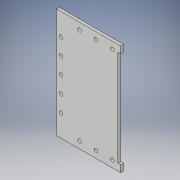
# Autodesk Inventor part: КВ33.000.103 - Стенка тонкая
Saved by Autodesk Inventor 2019 (Build 230136000, 136)
## iProperties
Created: 2021-04-18
Part Number: КВ33.000.103 - Стенка тонкая
Material: Типовые
Document SubType Name: Modeling
Designer: Петров Иван
Density: 1 g/cm^3
Appearance: По умолчанию
Author: Петров Иван
Autodesk Inventor part; units mm, degrees
ref_plane "YZ Plane" through (0, 0, 0) normal (1, 0, 0) x (0, 1, 0)
ref_plane "XZ Plane" through (0, 0, 0) normal (0, 1, 0) x (-1, 0, 0)
ref_plane "XY Plane" through (0, 0, 0) normal (0, 0, 1) x (1, 0, 0)
sketch "Sketch3" plane through (0, 0, 0) normal (0, 0, 1) x (1, 0, 0)
  circle A0 centre (51, -10.8228) radius 2 projected
  circle A1 centre (33, -10.8228) radius 2 projected
  circle A2 centre (15, -10.8228) radius 2 projected
  line L0 (0, -18.3228) -> (60, -18.3228) projected
  line L1 (0, -18.3228) -> (0, -13.3228) projected
  line L2 (10, -13.3228) -> (0, -13.3228) projected
  line L3 (10, -3.3228) -> (10, -13.3228) projected
  line L4 (10, -3.3228) -> (57, -3.3228) projected
  line L5 (60, -18.3228) -> (60, -10.8228) projected
  circle A3 centre (-5, 77.6772) radius 2 projected
  circle A4 centre (-5, 59.6772) radius 2 projected
  circle A5 centre (-5, 23.6772) radius 2 projected
  circle A6 centre (-5, 5.6772) radius 2 projected
  circle A7 centre (-5, 41.6772) radius 2 projected
  line L6 (-10, -18.3228) -> (-10, 101.6772) projected
  line L7 (-10, 101.6772) -> (0, 101.6772) projected
  line L8 (0, 96.6772) -> (0, 101.6772) projected
  line L9 (0, 96.6772) -> (10, 96.6772) projected
  line L10 (10, -13.3228) -> (10, 96.6772) projected
  line L11 (0, -13.3228) -> (10, -13.3228) projected
  line L12 (0, -18.3228) -> (0, -13.3228) projected
  line L13 (-10, -18.3228) -> (0, -18.3228) projected
  circle A8 centre (51, 94.1772) radius 2 projected
  circle A9 centre (33, 94.1772) radius 2 projected
  circle A10 centre (15, 94.1772) radius 2 projected
  line L14 (0, 101.6772) -> (60, 101.6772) projected
  line L15 (60, 94.1772) -> (60, 101.6772) projected
  line L16 (10, 86.6772) -> (57, 86.6772) projected
  line L17 (10, 96.6772) -> (10, 86.6772) projected
  line L18 (0, 96.6772) -> (10, 96.6772) projected
  line L19 (0, 101.6772) -> (0, 96.6772) projected
  line L20 (57, -10.8228) -> (60, -10.8228) projected
  line L21 (57, -3.3228) -> (57, -10.8228) projected
  line L22 (60, 94.1772) -> (57, 94.1772) projected
  line L23 (57, 94.1772) -> (57, 86.6772) projected
  line L24 (57, 86.6772) -> (57, -4.2516)
  point P0 (0, 0)
  constraints: 2 end point, 1 point on line
extrude "Extrusion2" add sketch "Sketch3" along normal blind 3
body "Solid2"
